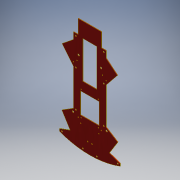
# Autodesk Inventor part: baseplate
Saved by Autodesk Inventor 2016 (Build 200138000, 138)
## iProperties
Created: 2016-09-22
Part Number: baseplate
Material: Nylon 6/6
Document SubType Name: Modeling
Designer: Jakub
Density: 1.13 g/cm^3
Appearance: Nylon 6
Mass: 17.2622 g
Surface Area: 319.515 cm^2
Volume: 15.2763 cm^3
Author: Jakub
Autodesk Inventor part; units mm, degrees
ref_plane "YZ Plane" through (0, 0, 0) normal (1, 0, 0) x (0, 1, 0)
ref_plane "XZ Plane" through (0, 0, 0) normal (0, 1, 0) x (-1, 0, 0)
ref_plane "XY Plane" through (0, 0, 0) normal (0, 0, 1) x (1, 0, 0)
sketch "Sketch1" plane through (0, 0, 0) normal (0, 1, 0) x (-1, 0, 0)
  circle A0 centre (0, 0) radius 165
  line L0 (35, 100) -> (-35, 100)
  line L1 (-35, 100) -> (-35, -100)
  line L2 (-35, -100) -> (35, -100)
  line L3 (35, -100) -> (35, 100)
  line L4 (35, 100) -> (-35, -100) construction
  line L5 (-35, 100) -> (35, -100) construction
  line L6 (35, -100) -> (65, -100)
  line L7 (-35, -100) -> (-65, -100)
  arc A1 (-65, -100) -> (65, -100) centre (0, 73.0722) ccw
  line L8 (120, 113.2475) -> (-120, -113.2475) construction
  line L9 (-120, 113.2475) -> (120, -113.2475) construction
  line L10 (35, -100) -> (35, -60)
  line L11 (-95, -134.9074) -> (95, 134.9074) construction
  line L12 (95, -134.9074) -> (-95, 134.9074) construction
  line L13 (65, -100) -> (65, -95)
  line L14 (65, -95) -> (35, -84.0809)
  line L15 (-65, -100) -> (-65, -95)
  line L16 (-65, -95) -> (-35, -84.0809)
  line L17 (35, -60) -> (51.961, -70.5984)
  line L18 (35, -60) -> (55, -60) construction
  line L19 (51.961, -70.5984) -> (41.9545, -86.6121)
  line L20 (51.961, -70.5984) -> (70.844, -70.5984) construction
  line L21 (51.961, -70.5984) -> (59.9098, -57.8777)
  line L22 (59.9098, -57.8777) -> (35, -42.3123)
  line L23 (-35, -100) -> (-35, -60)
  line L24 (-35, -60) -> (-51.961, -70.5984)
  line L25 (-35, -60) -> (-15, -60) construction
  line L26 (-51.961, -70.5984) -> (-41.9545, -86.6121)
  line L27 (-51.961, -70.5984) -> (-59.9098, -57.8777)
  line L28 (-59.9098, -57.8777) -> (-35, -42.3123)
  line L29 (-35, 100) -> (-35, 60)
  line L30 (35, 100) -> (35, 60)
  line L31 (-35, 60) -> (-47.5864, 75.5429)
  line L32 (-35, 60) -> (-15, 60) construction
  line L33 (35, 60) -> (47.5864, 75.5429)
  line L34 (35, 60) -> (55, 60) construction
  line L35 (47.5864, 75.5429) -> (35, 85.7352)
  line L36 (47.5864, 75.5429) -> (59.2436, 66.1031)
  line L37 (47.5864, 75.5429) -> (62.5864, 75.5429) construction
  line L38 (59.2436, 66.1031) -> (35, 36.1648)
  line L39 (35, 100) -> (35, 135)
  line L40 (35, 135) -> (20, 135)
  line L41 (20, 135) -> (20, 100)
  line L42 (-35, 100) -> (-35, 135)
  line L43 (-35, 135) -> (-20, 135)
  line L44 (-20, 135) -> (-20, 100)
  line L45 (-59.2436, 66.1031) -> (-20.7201, 66.1031) construction
  line L46 (-47.5864, 75.5429) -> (-35, 85.7352)
  line L47 (-47.5864, 75.5429) -> (-31.3907, 75.5429) construction
  line L48 (-47.5864, 75.5429) -> (-59.2436, 66.1031)
  line L49 (-47.5864, 75.5429) -> (-32.5864, 75.5429) construction
  line L50 (-59.2436, 66.1031) -> (-35, 36.1648)
  dimension "d0" = 330
  dimension "d2" = 70
  dimension "d3" = 200
  dimension "d4" = 30
  dimension "d5" = 30
  dimension "d6" = 240
  dimension "d8" = 40
  dimension "d9" = 190
  dimension "d10" = 5
  dimension "d11" = 110
  dimension "d12" = 5
  dimension "d13" = 110
  dimension "d14" = 20
  dimension "d15" = 32
  dimension "d16" = 122
  dimension "d17" = 15
  dimension "d18" = 40
  dimension "d19" = 20
  dimension "d20" = 148
  dimension "d21" = 90
  dimension "d22" = 15
  dimension "d23" = 40
  dimension "d24" = 40
  dimension "d25" = 20
  dimension "d26" = 129
  dimension "d29" = 20
  dimension "d30" = 51
  dimension "d31" = 15
  dimension "d32" = 39
  dimension "d33" = 90
  dimension "d34" = 35
  dimension "d35" = 15
  dimension "d36" = 90
  dimension "d37" = 35
  dimension "d38" = 15
  dimension "d39" = 90
  dimension "d41" = 39
  dimension "d42" = 15
  dimension "d43" = 141
  dimension "d44" = 90
  constraints: 102 end point, 16 point on line, 12 horizontal, 10 perpendicular, 8 equal length, 6 midpoint, 4 point on circle, 2 centre point, 2 parallel, 1 coincident, 1 vertical
  measures "d0" diameter of A0
  measures "d2" distance of L2.end L1.end
  measures "d3" distance of L1.end L0.end
  measures "d4" distance of L2.end L6.end
  measures "d5" distance of L1.end L7.end
  measures "d6" distance of L9.end L8.end
  measures "d8" distance of L2.end L10.end
  measures "d9" distance of L12.end L11.end
  measures "d10" distance of L6.end L13.end
  measures "d11" angle of L14 L13
  measures "d12" distance of L7.end L15.end
  measures "d13" angle of L15 L16
  measures "d14" distance of L10.end L17.end
  measures "d15" angle of L17 L18
  measures "d16" angle of L19 L20
  measures "d17" distance of L17.end L21.end
  measures "d18" distance of L1.end L23.end
  measures "d19" distance of L23.end L24.end
  measures "d20" angle of L24 L25
  measures "d21" angle of L26 L24
  measures "d22" distance of L24.end L27.end
  measures "d23" distance of L0.end L29.end
  measures "d24" distance of L0.start L30.end
  measures "d25" distance of L29.end L31.end
  measures "d26" angle of L32 L31
  measures "d29" distance of L30.end L33.end
  measures "d30" angle of L34 L33
  measures "d31" distance of L33.end L36.end
  measures "d32" angle of L36 L37
  measures "d33" angle of L36 L38
  measures "d34" distance of L0.start L39.end
  measures "d35" distance of L39.end L40.end
  measures "d36" angle of L40 L39
  measures "d37" distance of L0.end L42.end
  measures "d38" distance of L42.end L43.end
  measures "d39" angle of L42 L43
  measures "d41" angle of L47 L46
  measures "d42" distance of L31.end L45.start
  measures "d43" angle of L48 L49
  measures "d44" angle of L50 L48
extrude "Extrusion1" add sketch "Sketch1" along normal blind 1 contours L3 L2 L1 L0 | L0 L41 L40 L39 | L35 L33 L3 | L0 L42 L43 L44 | L33 L36 L38 L3 | L1 L31 L46 | L22 L21 L17 L3 | L1 L50 L48 L31 | L17 L19 L14 L3 | L14 L13 L6 L3 | L1 L24 L27 L28 | L6 A1 L7 L2 | L1 L16 L26 L24 | L7 L15 L16 L1
sketch "Sketch2" plane through (0, 1, 0) normal (0, 1, 0) x (1, 0, 0)
  line L0 (-59.9098, 57.8777) -> (-35, 42.3123) projected
  line L1 (-59.9098, 57.8777) -> (-51.961, 70.5984)
  line L2 (-41.9545, 86.6121) -> (-59.9098, 57.8777) projected
  line L3 (-51.961, 70.5984) -> (-30.7598, 57.3504)
  line L4 (-30.7598, 57.3504) -> (-36.059, 48.8699)
  line L5 (-30.7598, 57.3504) -> (-20.7598, 57.3504) construction
  circle A0 centre (-36.059, 48.8699) radius 2
  line L6 (35, 42.3123) -> (59.9098, 57.8777) projected
  line L7 (59.9098, 57.8777) -> (51.961, 70.5984)
  line L8 (59.9098, 57.8777) -> (41.9545, 86.6121) projected
  line L9 (51.961, 70.5984) -> (30.7598, 57.3504)
  line L10 (30.7598, 57.3504) -> (36.059, 48.8699)
  circle A1 centre (36.059, 48.8699) radius 2
  line L11 (35, -85.7352) -> (59.2436, -66.1031) projected
  line L12 (59.2436, -66.1031) -> (47.5864, -75.5429)
  line L13 (59.2436, -66.1031) -> (74.2436, -66.1031) construction
  line L14 (47.5864, -75.5429) -> (31.8534, -56.1143)
  line L15 (31.8534, -56.1143) -> (24.0819, -62.4075)
  circle A2 centre (24.0819, -62.4075) radius 2
  line L16 (-59.2436, -66.1031) -> (-35, -85.7352) projected
  line L17 (-59.2436, -66.1031) -> (-47.5864, -75.5429)
  line L18 (-59.2436, -66.1031) -> (-44.2436, -66.1031) construction
  line L19 (-47.5864, -75.5429) -> (-31.8534, -56.1143)
  line L20 (-31.8534, -56.1143) -> (-24.0819, -62.4075)
  circle A3 centre (-24.0819, -62.4075) radius 2
  point P0 (0, 0)
  dimension "d47" = 15
  dimension "d48" = 25
  dimension "d49" = 10
  dimension "d50" = 122
  dimension "d51" = 4
  dimension "d52" = 15
  dimension "d53" = 25
  dimension "d54" = 90
  dimension "d55" = 10
  dimension "d56" = 90
  dimension "d57" = 4
  dimension "d58" = 15
  dimension "d59" = 141
  dimension "d60" = 25
  dimension "d61" = 90
  dimension "d62" = 10
  dimension "d63" = 90
  dimension "d64" = 4
  dimension "d65" = 15
  dimension "d66" = 39
  dimension "d67" = 25
  dimension "d68" = 90
  dimension "d69" = 10
  dimension "d70" = 90
  dimension "d71" = 4
  constraints: 30 end point, 7 perpendicular, 4 centre point, 4 coincident, 3 equal length, 3 horizontal, 2 collinear, 2 point on line
  measures "d47" distance of L0.start L1.end
  measures "d48" distance of L1.end L3.end
  measures "d49" distance of L3.end L4.end
  measures "d50" angle of L4 L5
  measures "d51" diameter of A0
  measures "d52" distance of L6.end L7.end
  measures "d53" distance of L7.end L9.end
  measures "d54" angle of L9 L7
  measures "d55" distance of L9.end L10.end
  measures "d56" angle of L10 L9
  measures "d57" diameter of A1
  measures "d58" distance of L11.end L12.end
  measures "d59" angle of L12 L13
  measures "d60" distance of L12.end L14.end
  measures "d61" angle of L12 L14
  measures "d62" distance of L14.end L15.end
  measures "d63" angle of L15 L14
  measures "d64" diameter of A2
  measures "d65" distance of L16.start L17.end
  measures "d66" angle of L17 L18
  measures "d67" distance of L17.end L19.end
  measures "d68" angle of L19 L17
  measures "d69" distance of L19.end L20.end
  measures "d70" angle of L19 L20
  measures "d71" diameter of A3
extrude "Extrusion2" cut sketch "Sketch2" against normal up to next
sketch "Sketch3" plane through (0, 1, 0) normal (0, 1, 0) x (1, 0, 0)
  line L0 (59.2436, -66.1031) -> (35, -36.1648) projected
  line L1 (59.2436, -66.1031) -> (40.9933, -43.5659)
  line L2 (40.9933, -43.5659) -> (39.1053, -41.2344)
  line L3 (39.1053, -41.2344) -> (35.2196, -44.381)
  line L4 (35.2196, -44.381) -> (27.4482, -50.6742)
  circle A0 centre (27.4482, -50.6742) radius 1
  circle A1 centre (35.2196, -44.381) radius 1
  point P0 (0, 0)
  dimension "d74" = 29
  dimension "d75" = 3
  dimension "d76" = 5
  dimension "d77" = 10
  dimension "d78" = 2
  dimension "d79" = 2
  constraints: 8 end point, 3 point on line, 2 centre point, 2 coincident, 1 perpendicular
  measures "d74" distance of L0.start L1.end
  measures "d75" distance of L1.end L2.end
  measures "d76" distance of L2.end L3.end
  measures "d77" distance of L3.end L4.end
  measures "d78" diameter of A0
  measures "d79" diameter of A1
extrude "Extrusion3" cut sketch "Sketch3" against normal up to next
sketch "Sketch4" plane through (0, 1, 0) normal (0, 1, 0) x (1, 0, 0)
  line L0 (-59.2436, -66.1031) -> (-35, -85.7352) projected
  line L1 (-59.2436, -66.1031) -> (-39.1053, -41.2344)
  line L2 (-35, -36.1648) -> (-59.2436, -66.1031) projected
  line L3 (-39.1053, -41.2344) -> (-35.2196, -44.381)
  line L4 (-35.2196, -44.381) -> (-27.4482, -50.6742)
  circle A0 centre (-35.2196, -44.381) radius 1
  circle A1 centre (-27.4482, -50.6742) radius 1
  point P0 (0, 0)
  dimension "d82" = 32
  dimension "d83" = 5
  dimension "d84" = 90
  dimension "d85" = 10
  dimension "d86" = 180
  dimension "d87" = 2
  dimension "d88" = 2
  constraints: 6 end point, 2 centre point, 2 coincident, 1 collinear, 1 perpendicular, 1 point on line
  measures "d82" distance of L0.start L1.end
  measures "d83" distance of L1.end L3.end
  measures "d84" angle of L1 L3
  measures "d85" distance of L3.end L4.end
  measures "d86" angle of L4 L3
  measures "d87" diameter of A0
  measures "d88" diameter of A1
extrude "Extrusion4" cut sketch "Sketch4" against normal up to next
sketch "Sketch5" plane through (0, 1, 0) normal (0, 1, 0) x (1, 0, 0)
  line L0 (59.9098, 57.8777) -> (41.9545, 86.6121) projected
  line L1 (59.9098, 57.8777) -> (44.0122, 83.3191)
  line L2 (59.9098, 57.8777) -> (89.9098, 57.8777) construction
  line L3 (44.0122, 83.3191) -> (16.8746, 66.3617)
  line L4 (16.8746, 66.3617) -> (19.5242, 62.1214)
  line L5 (19.5242, 62.1214) -> (24.8234, 53.641)
  circle A0 centre (19.5242, 62.1214) radius 1
  circle A1 centre (24.8234, 53.641) radius 1
  point P0 (0, 0)
  dimension "d91" = 30
  dimension "d92" = 122
  dimension "d93" = 32
  dimension "d94" = 90
  dimension "d95" = 5
  dimension "d96" = 10
  dimension "d97" = 2
  dimension "d98" = 2
  constraints: 10 end point, 2 centre point, 2 coincident, 2 perpendicular, 1 collinear, 1 equal length, 1 horizontal, 1 point on line
  measures "d91" distance of L0.start L1.end
  measures "d92" angle of L2 L1
  measures "d93" distance of L1.end L3.end
  measures "d94" angle of L3 L1
  measures "d95" distance of L3.end L4.end
  measures "d96" distance of L4.end L5.end
  measures "d97" diameter of A0
  measures "d98" diameter of A1
extrude "Extrusion5" cut sketch "Sketch5" against normal up to next
sketch "Sketch6" plane through (0, 1, 0) normal (0, 1, 0) x (1, 0, 0)
  line L0 (-41.9545, 86.6121) -> (-59.9098, 57.8777) projected
  line L1 (-59.9098, 57.8777) -> (-44.0122, 83.3191)
  line L2 (-44.0122, 83.3191) -> (-16.8746, 66.3617)
  line L3 (-44.0122, 83.3191) -> (-12.0122, 83.3191) construction
  line L4 (-16.8746, 66.3617) -> (-19.5242, 62.1214)
  line L5 (-19.5242, 62.1214) -> (-24.8234, 53.641)
  circle A0 centre (-24.8234, 53.641) radius 1
  circle A1 centre (-19.5242, 62.1214) radius 1
  point P0 (0, 0)
  dimension "d101" = 30
  dimension "d106" = 32
  dimension "d107" = 32
  dimension "d108" = 5
  dimension "d109" = 10
  dimension "d110" = 2
  dimension "d111" = 2
  constraints: 10 end point, 2 centre point, 2 coincident, 1 equal length, 1 horizontal, 1 perpendicular, 1 point on line
  measures "d101" distance of L0.end L1.end
  measures "d106" distance of L1.end L2.end
  measures "d107" angle of L2 L3
  measures "d108" distance of L2.end L4.end
  measures "d109" distance of L4.end L5.end
  measures "d110" diameter of A0
  measures "d111" diameter of A1
extrude "Extrusion6" cut sketch "Sketch6" against normal up to next
sketch "Sketch7" plane through (0, 1, 0) normal (0, 1, 0) x (1, 0, 0)
  line L0 (-35, 42.3123) -> (-35, -36.1648) projected
  line L1 (-35, 42.3123) -> (-30, 42.3123)
  line L2 (35, -36.1648) -> (35, 42.3123) projected
  line L3 (35, 42.3123) -> (30, 42.3123)
  circle A0 centre (-30, 42.3123) radius 1.5
  circle A1 centre (30, 42.3123) radius 1.5
  point P0 (0, 0)
  dimension "d114" = 5
  dimension "d115" = 5
  dimension "d116" = 3
  dimension "d117" = 3
  constraints: 4 end point, 2 centre point, 2 coincident, 2 horizontal
  measures "d114" distance of L0.start L1.end
  measures "d115" distance of L2.end L3.end
  measures "d116" diameter of A0
  measures "d117" diameter of A1
extrude "Extrusion7" cut sketch "Sketch7" against normal through all
sketch "Sketch8" plane through (0, 1, 0) normal (0, 1, 0) x (1, 0, 0)
  arc A0 (65, 100) -> (-65, 100) centre (0, -73.0722) ccw projected
  line L0 (0, 111.8034) -> (0, 106.8034)
  line L1 (0, 106.8034) -> (-15, 106.8034)
  line L2 (0, 106.8034) -> (15, 106.8034)
  circle A1 centre (-15, 106.8034) radius 1.5
  circle A2 centre (15, 106.8034) radius 1.5
  line L3 (-65, 100) -> (-65, 95) projected
  line L4 (-65, 97.5) -> (-60, 97.5)
  line L5 (65, 95) -> (65, 100) projected
  line L6 (65, 97.5) -> (60, 97.5)
  circle A3 centre (-60, 97.5) radius 1.5
  circle A4 centre (60, 97.5) radius 1.5
  point P0 (0, 0)
  dimension "d120" = 5
  dimension "d121" = 15
  dimension "d122" = 15
  dimension "d123" = 3
  dimension "d124" = 3
  dimension "d125" = 5
  dimension "d126" = 5
  dimension "d127" = 3
  dimension "d128" = 3
  constraints: 10 end point, 4 centre point, 4 coincident, 4 horizontal, 2 midpoint, 1 point on circle, 1 vertical
  measures "d120" distance of L0.start L0.end
  measures "d121" distance of L0.end L1.end
  measures "d122" distance of L0.end L2.end
  measures "d123" diameter of A1
  measures "d124" diameter of A2
  measures "d125" distance of L4.start L4.end
  measures "d126" distance of L6.start L6.end
  measures "d127" diameter of A3
  measures "d128" diameter of A4
extrude "Extrusion8" cut sketch "Sketch8" against normal through all
sketch "Sketch9" plane through (0, 1, 0) normal (0, 1, 0) x (1, 0, 0)
  line L0 (-35, -135) -> (-20, -135) projected
  line L1 (-20, -100) -> (20, -100) projected
  line L2 (-35, -135) -> (-20, -135)
  line L3 (-20, -135) -> (-20, -100)
  line L4 (-20, -100) -> (-35, -100)
  line L5 (-35, -100) -> (-35, -135)
  line L6 (35, -135) -> (35, -85.7352) projected
  line L7 (20, -100) -> (35, -100)
  line L8 (35, -100) -> (35, -135)
  line L9 (35, -135) -> (20, -135)
  line L10 (20, -135) -> (20, -100)
  point P0 (0, 0)
  constraints: 16 end point, 4 parallel, 2 horizontal, 2 perpendicular
extrude "Extrusion9" cut sketch "Sketch9" against normal up to next
sketch "Sketch10" plane through (0, 1, 0) normal (0, 1, 0) x (1, 0, 0)
  line L0 (-35, -36.1648) -> (-30, -36.1648)
  line L1 (35, -36.1648) -> (35, 42.3123) projected
  line L2 (35, -36.1648) -> (30, -36.1648)
  line L3 (35, -100) -> (35, -85.7352) projected
  line L4 (35, -100) -> (30, -100)
  line L5 (30, -100) -> (30, -95)
  line L6 (30, -95) -> (35, -95)
  line L7 (35, -95) -> (35, -100)
  line L8 (-35, -85.7352) -> (-35, -100) projected
  line L9 (-35, -100) -> (-30, -100)
  line L10 (-30, -100) -> (-30, -95)
  line L11 (-30, -95) -> (-35, -95)
  line L12 (-35, -95) -> (-35, -100)
  circle A0 centre (-30, -95) radius 1.5
  circle A1 centre (30, -95) radius 1.5
  circle A2 centre (30, -36.1648) radius 1.5
  circle A3 centre (-30, -36.1648) radius 1.5
  point P0 (0, 0)
  dimension "d133" = 5
  dimension "d134" = 5
  dimension "d135" = 5
  dimension "d136" = 5
  dimension "d137" = 5
  dimension "d138" = 5
  dimension "d139" = 3
  dimension "d140" = 3
  dimension "d141" = 3
  dimension "d142" = 3
  constraints: 20 end point, 4 centre point, 4 coincident, 4 horizontal, 4 parallel, 2 perpendicular
  measures "d133" distance of L0.start L0.end
  measures "d134" distance of L1.start L2.end
  measures "d135" distance of L5.end L6.end
  measures "d136" distance of L4.end L5.end
  measures "d137" distance of L11.end L10.end
  measures "d138" distance of L10.end L9.end
  measures "d139" diameter of A0
  measures "d140" diameter of A1
  measures "d141" diameter of A2
  measures "d142" diameter of A3
extrude "Extrusion10" cut sketch "Sketch10" against normal through all contours A1 L5 L6 | L6 L5 A1 | A0 L10 L11 | L11 L10 A0 | A2 | A3
sketch "Sketch12" plane through (0, 0, 0) normal (0, -1, 0) x (1, 0, 0)
  line L0 (-18.5, 1.5) -> (18.5, 1.5)
  line L1 (18.5, 1.5) -> (18.5, -51.5)
  line L2 (18.5, -51.5) -> (-18.5, -51.5)
  line L3 (-18.5, -51.5) -> (-18.5, 1.5)
  line L4 (-18.5, 1.5) -> (18.5, -51.5) construction
  line L5 (18.5, 1.5) -> (-18.5, -51.5) construction
  circle A0 centre (18.5, 1.5) radius 1
  circle A1 centre (18.5, -51.5) radius 1
  circle A2 centre (-18.5, -51.5) radius 1
  circle A3 centre (-18.5, 1.5) radius 1
  point P0 (0, 0)
  point P1 (0, -25)
  dimension "d152" = 37
  dimension "d153" = 53
  dimension "d154" = 25
  dimension "d155" = 2
  dimension "d156" = 2
  dimension "d157" = 2
  dimension "d158" = 2
  constraints: 12 end point, 4 centre point, 4 coincident, 2 midpoint, 2 parallel, 1 horizontal, 1 perpendicular
  measures "d152" distance of L1.end L2.end
  measures "d153" distance of L0.end L1.end
  measures "d154" distance of point (0, 0) point (0, -25)
  measures "d155" diameter of A0
  measures "d156" diameter of A1
  measures "d157" diameter of A2
  measures "d158" diameter of A3
extrude "Extrusion12" cut sketch "Sketch12" against normal up to next contours L3 A3 L0 | L0 A3 L3 | A0 L1 L0 | L0 L1 A0 | A2 L2 L3 | L3 L2 A2 | A1 L2 L1 | L1 L2 A1
sketch "Sketch13" plane through (0, 0, 0) normal (0, -1, 0) x (1, 0, 0)
  arc A0 (-65, -100) -> (65, -100) centre (0, 73.0722) ccw projected
  line L0 (0, -111.8034) -> (0, -88.8034)
  line L1 (0, -88.8034) -> (4.5, -88.8034)
  line L2 (0, -88.8034) -> (-4.5, -88.8034)
  circle A1 centre (4.5, -88.8034) radius 1.25
  circle A2 centre (-4.5, -88.8034) radius 1.25
  point P0 (0, 0)
  dimension "d161" = 23
  dimension "d162" = 4.5
  dimension "d163" = 4.5
  dimension "d164" = 2.5
  dimension "d165" = 2.5
  constraints: 6 end point, 2 centre point, 2 coincident, 1 horizontal, 1 perpendicular, 1 point on circle, 1 vertical
  measures "d161" distance of L0.start L0.end
  measures "d162" distance of L0.end L1.end
  measures "d163" distance of L0.end L2.end
  measures "d164" diameter of A1
  measures "d165" diameter of A2
extrude "Extrusion13" cut sketch "Sketch13" against normal up to next
sketch "Sketch14" plane through (0, 1, 0) normal (0, 1, 0) x (1, 0, 0)
  line L0 (-35, -85.7352) -> (-35, -100) projected
  line L1 (-35, -100) -> (-25, -100)
  line L2 (35, -100) -> (-35, -100) projected
  line L3 (-25, -100) -> (25, -100)
  line L4 (25, -100) -> (25, -130)
  line L5 (25, -130) -> (-25, -130)
  line L6 (-25, -130) -> (-25, -100)
  point P0 (0, 0)
  dimension "d168" = 10
  dimension "d169" = 50
  dimension "d170" = 30
  constraints: 10 end point, 2 parallel, 1 horizontal, 1 perpendicular, 1 point on line
  measures "d168" distance of L0.end L1.end
  measures "d169" distance of L4.end L5.end
  measures "d170" distance of L3.end L4.end
extrude "Extrusion14" add sketch "Sketch14" against normal blind 1
sketch "Sketch15" plane through (0, 1, 0) normal (0, 1, 0) x (1, 0, 0)
  line L0 (-20, 47.0842) -> (20, 47.0842)
  line L1 (20, 47.0842) -> (20, 2.0842)
  line L2 (20, 2.0842) -> (-20, 2.0842)
  line L3 (-20, 2.0842) -> (-20, 47.0842)
  line L4 (-20, 47.0842) -> (20, 2.0842) construction
  line L5 (20, 47.0842) -> (-20, 2.0842) construction
  line L6 (-15, -17.8571) -> (15, -17.8571)
  line L7 (15, -17.8571) -> (15, -97.8571)
  line L8 (15, -97.8571) -> (-15, -97.8571)
  line L9 (-15, -97.8571) -> (-15, -17.8571)
  line L10 (-15, -17.8571) -> (15, -97.8571) construction
  line L11 (15, -17.8571) -> (-15, -97.8571) construction
  point P0 (0, 0)
  point P1 (0, 24.5842)
  point P2 (0, -57.8571)
  dimension "d173" = 40
  dimension "d174" = 45
  dimension "d175" = 30
  dimension "d176" = 80
  constraints: 24 end point, 4 midpoint, 4 parallel, 2 horizontal, 2 perpendicular
  measures "d173" distance of L1.end L2.end
  measures "d174" distance of L0.end L1.end
  measures "d175" distance of L7.end L8.end
  measures "d176" distance of L6.end L7.end
extrude "Extrusion15" cut sketch "Sketch15" against normal up to next
body "Solid1"
